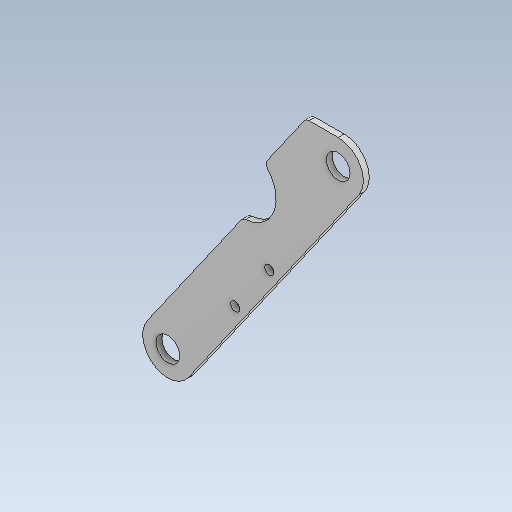
# Autodesk Inventor part: BackLink_frame
Saved by Autodesk Inventor 2020.4 (Build 244396000, 396)
## iProperties
Created: 2021-10-03
Part Number: BackLink_frame
Material: GFRP
Document SubType Name: Modeling
Designer: Masato Kubotera
Density: 1.75 g/cm^3
Appearance: 滑らか - 淡い灰色
Author: Masato Kubotera
Autodesk Inventor part; units mm, degrees
ref_plane "YZ Plane" through (0, 0, 0) normal (1, 0, 0) x (0, 1, 0)
ref_plane "XZ Plane" through (0, 0, 0) normal (0, 1, 0) x (-1, 0, 0)
ref_plane "XY Plane" through (0, 0, 0) normal (0, 0, 1) x (1, 0, 0)
derived "Link_basis.ipt"
sketch "スケッチ1" plane through (0, 0, 0) normal (0, 0, 1) x (1, 0, 0)
  circle A0 centre (0, 0) radius 6
  circle A1 centre (-57.3576, -81.9152) radius 4
  arc A2 (-64.2795, -77.0685) -> (-57.3576, -90.3652) centre (-57.3576, -81.9152) ccw
  arc A3 (-0.1434, -10.9991) -> (-4.8354, 9.8802) centre (0, 0) ccw
  line L0 (-58.3761, -41.5269) -> (-32.5651, -4.6651) construction
  line L1 (-32.5651, -4.6651) -> (-28.4694, -7.533) construction
  line L2 (-28.4694, -7.533) -> (-54.2803, -44.3948) construction
  line L3 (-54.2803, -44.3948) -> (-58.3761, -41.5269) construction
  line L4 (-58.3761, -41.5269) -> (-28.4694, -7.533) construction
  line L5 (-32.5651, -4.6651) -> (-54.2803, -44.3948) construction
  line L6 (-56.3282, -42.9609) -> (-30.5172, -6.099) construction
  circle A4 centre (-54.8942, -40.913) radius 1.55
  circle A5 centre (-43.4227, -24.5299) radius 1.55
  line L7 (-45.4706, -23.096) -> (-41.3748, -25.9639) construction
  circle A6 centre (-31.9512, -8.1469) radius 1.55
  line L8 (-59.1952, -40.9534) -> (-33.3843, -4.0915)
  line L9 (-33.3843, -4.0915) -> (-4.8354, 9.8802)
  line L10 (-59.1952, -40.9534) -> (-62.8179, -74.9812)
  line L11 (-62.8179, -74.9812) -> (-64.2795, -77.0685)
  line L12 (-32.3614, -57.0111) -> (-0.1434, -10.9991)
  line L13 (0, 0) -> (32, 0) construction
  line L14 (32, 0) -> (32, 20) construction
  circle A7 centre (32, 20) radius 4
  arc A8 (38.9218, 15.1533) -> (32, 28.45) centre (32, 20) ccw
  line L15 (32, 20) -> (32, 37) construction
  circle A9 centre (32, 37) radius 4 construction
  circle A10 centre (32, 37) radius 8.45 construction
  line L16 (-57.3576, -81.9152) -> (0, 0) construction
  circle A11 centre (0, 0) radius 8.5 construction
  line L17 (0, 0) -> (4.8754, 6.9628) construction
  circle A12 centre (4.8754, 6.9628) radius 1.35
  circle A13 centre (32, 20) radius 8 construction
  circle A14 centre (-57.3576, -81.9152) radius 8 construction
  line L18 (-50.4358, -86.7619) -> (-33.8321, -63.0494)
  line L19 (38.9218, 15.1533) -> (-18.4358, -66.7619)
  line L20 (32, 20) -> (-25.3576, -61.9152) construction
  circle A15 centre (-25.3576, -61.9152) radius 4
  circle A16 centre (-25.3576, -61.9152) radius 8 construction
  arc A17 (-0.0917, -11.0996) -> (7.185, 8.4608) centre (0, 0) ccw
  line L21 (25.0782, 24.8467) -> (10.3989, 3.8825)
  line L22 (-0.0917, -11.0996) -> (-32.2795, -57.0685)
  arc A18 (-32.2795, -57.0685) -> (-18.4358, -66.7619) centre (-25.3576, -61.9152) ccw
  arc A19 (-32.3614, -57.0111) -> (-32.5799, -66.4914) centre (-25.3576, -61.9152) ccw
  line L23 (-6.9628, 4.8754) -> (0, 0) construction
  circle A20 centre (-6.9628, 4.8754) radius 1.35
  circle A21 centre (-4.8754, -6.9628) radius 1.35
  circle A22 centre (6.9628, -4.8754) radius 1.35
  line L24 (-6.1434, -38.7459) -> (8.196, -18.2671) construction
  line L25 (8.196, -18.2671) -> (12.2917, -21.135) construction
  line L26 (12.2917, -21.135) -> (-2.0477, -41.6138) construction
  line L27 (-2.0477, -41.6138) -> (-6.1434, -38.7459) construction
  line L28 (-6.1434, -38.7459) -> (12.2917, -21.135) construction
  line L29 (8.196, -18.2671) -> (-2.0477, -41.6138) construction
  line L30 (10.2439, -19.701) -> (-4.0955, -40.1798) construction
  line L31 (1.0263, -28.5065) -> (5.122, -31.3744) construction
  circle A23 centre (8.8099, -21.7489) radius 1.55
  circle A24 centre (-2.6616, -38.132) radius 1.55
  line L32 (7.185, 8.4608) -> (21.1816, 28.45)
  line L33 (32, 28.45) -> (21.1816, 28.45)
  arc A25 (32, 28.45) -> (25.0782, 24.8467) centre (32, 20) ccw construction
  line L34 (-32.5799, -66.4914) -> (-49.2965, -90.3652)
  line L35 (-57.3576, -90.3652) -> (-49.2965, -90.3652)
  arc A26 (-57.3576, -90.3652) -> (-50.4358, -86.7619) centre (-57.3576, -81.9152) ccw construction
  point P0 (3.0742, -29.9404)
extrude "押し出し1" add sketch "スケッチ1" along normal blind 2 contours L19 A18 L22 A17 L32 L33 A8
fillet "フィレット1" radius 2 3 edges at (-0.0917, -11.0996, 1) (21.1816, 28.45, 1) (7.185, 8.4608, 1)
